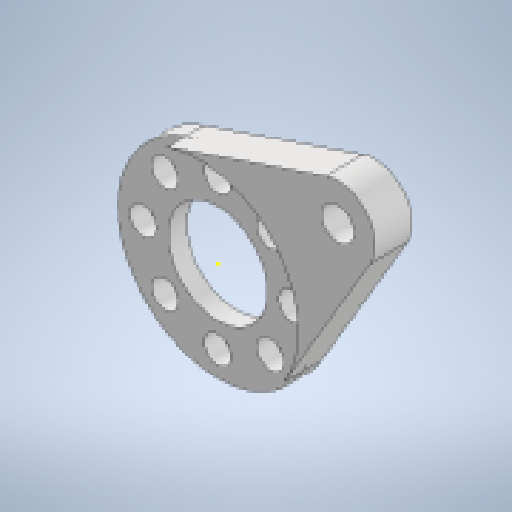
# Autodesk Inventor part: namida
Saved by Autodesk Inventor 2025.1 (Build 291241000, 241)
## iProperties
Created: 2024-09-01
Part Number: namida
Material: 一般
Document SubType Name: Modeling
Designer: right
Density: 1 g/cm^3
Appearance: 既定
Author: right
Autodesk Inventor part; units mm, degrees
ref_plane "YZ Plane" through (0, 0, 0) normal (1, 0, 0) x (0, 1, 0)
ref_plane "XZ Plane" through (0, 0, 0) normal (0, 1, 0) x (-1, 0, 0)
ref_plane "XY Plane" through (0, 0, 0) normal (0, 0, 1) x (1, 0, 0)
sketch "スケッチ1" plane through (0, 0, 0) normal (0, 0, 1) x (1, 0, 0)
  circle A0 centre (0, 0) radius 4
  circle A1 centre (0, 0) radius 8
  circle A2 centre (0, 0) radius 6 construction
  circle A3 centre (0, 6) radius 1.1
  circle A4 centre (-4.2426, 4.2426) radius 1.1
  circle A5 centre (-6, 0) radius 1.1
  circle A6 centre (-4.2426, -4.2426) radius 1.1
  circle A7 centre (0, -6) radius 1.1
  circle A8 centre (4.2426, -4.2426) radius 1.1
  circle A9 centre (6, 0) radius 1.1
  circle A10 centre (4.2426, 4.2426) radius 1.1
  dimension "d2" = 12
  dimension "d0" = 8
  dimension "d1" = 16
  dimension "d3" = 2.2
  dimension "d6" = 360
  constraints: 10 centre point, 3 coincident, 2 vertical alignment, 19 other
  measures "d0" diameter of A0
  measures "d1" diameter of A1
  measures "d3" diameter of A3
extrude "押し出し1" add sketch "スケッチ1" along normal blind 1.5
sketch "スケッチ2" plane through (0, 0, 0) normal (0, 0, -1) x (-1, 0, 0)
  circle A0 centre (-12.8215, -6.6226) radius 1.3
  circle A1 centre (-12.8215, -6.6226) radius 3
  circle A2 centre (0, 0) radius 8 projected
  line L0 (-15.0365, -4.5993) -> (-5.9067, 5.3955)
  line L1 (-12.4536, -9.5999) -> (0.9812, -7.9396)
  circle A3 centre (-4.758, 14.0841) radius 3 projected
  circle A4 centre (-12.8215, -6.6226) radius 1.3 construction
  dimension "d10" = 2.6
  dimension "d11" = 6
  constraints: 4 end point, 4 point on circle, 4 tangent, 2 centre point, 2 coincident
  measures "d10" diameter of A0
  measures "d11" diameter of A1
extrude "押し出し2" add sketch "スケッチ2" against normal blind 3 contours A1 | A1 L0 A2 L1
sketch "スケッチ3" plane through (0, 0, 1.5) normal (0, 0, 1) x (1, 0, 0)
  point P0 (0, 0)
